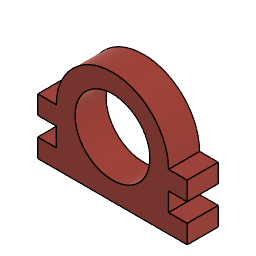
BarrelJackMount_v1 (Autodesk Fusion 360 design; units mm, degrees)
Autodesk Fusion 360 part; units mm, degrees
sketch "Sketch1" plane through (0, 0, 0) normal (0, 1, 0) x (1, 0, 0)
  line L0 (9, 1.5) -> (-9, 1.5) construction
  line L1 (-9, 1.5) -> (-9, -1.5) construction
  line L2 (9, -1.5) -> (9, 1.5) construction
  line L3 (9, 1.5) -> (-9, -1.5) construction
  line L4 (-9, 1.5) -> (9, -1.5) construction
  circle A0 centre (0, -4.5) radius 6
  circle A1 centre (0, -4.5) radius 9
  line L5 (0, 1.5) -> (0, 4.5) construction
  line L6 (0, 0) -> (0, -4.5) construction
  line L7 (-9, 1.5) -> (-9, -1.5)
  line L8 (-9, 1.5) -> (-6.7082, 1.5)
  line L9 (-9, -1.5) -> (-9, -4.5)
  line L10 (6.7082, 1.5) -> (9, 1.5)
  line L11 (9, 1.5) -> (9, -4.5)
  line L12 (-9, -1.5) -> (-12, -1.5)
  line L13 (-12, -1.5) -> (-12, -4.5)
  line L14 (-12, -4.5) -> (-9, -4.5)
  line L15 (-9, 1.5) -> (-12, 1.5)
  line L16 (-12, 1.5) -> (-12, 4.5)
  line L17 (9, 1.5) -> (12, 1.5)
  line L18 (12, 1.5) -> (12, 4.5)
  line L19 (12, 4.5) -> (-12, 4.5)
  line L20 (9, -4.5) -> (12, -4.5)
  line L21 (12, -4.5) -> (12, -1.5)
  line L22 (12, -1.5) -> (9, -1.5)
  dimension "d1" = 18
  dimension "d2" = 3
  dimension "d3" = 12
  dimension "d4" = 18
  dimension "d5" = 3
  dimension "d6" = 3
  dimension "d7" = 3
  dimension "d8" = 3
  dimension "d9" = 3
  dimension "d10" = 3
  dimension "d11" = 3
  dimension "d12" = 3
  dimension "d13" = 3
  constraint horizontal L0
  constraint perpendicular L0 L1
  constraint parallel L1 L2
  constraint coincident L3 L6.start
  constraint coincident L4 L6.start
  constraint coincident L6.start origin
  constraint concentric A0 A1
  constraint midpoint L0 L5.start
  constraint perpendicular L0 L5
  constraint coincident A1 L5.end
  constraint coincident A0.centre A1.centre
  constraint vertical L6
  constraint coincident A1 L8.end
  constraint coincident L0 L8.end
  constraint coincident A1 L9.end
  constraint tangent A1 L9
  constraint coincident A1 L10.start
  constraint coincident L0 L10.start
  constraint coincident A1 L11.end
  constraint tangent A1 L11
  constraint perpendicular L9 L12
  constraint perpendicular L12 L13
  constraint perpendicular L9 L14
  constraint perpendicular L1 L15
  constraint perpendicular L15 L16
  constraint perpendicular L2 L17
  constraint perpendicular L17 L18
  constraint perpendicular L11 L20
  constraint perpendicular L20 L21
  measures "d1" distance of L1.end L2.start
  measures "d2" distance of L0.end L1.end
  measures "d3" diameter of A0
  measures "d4" diameter of A1
  measures "d5" distance of L5.start L5.end
  measures "d6" distance of L1.end L12.end
  measures "d7" distance of L12.end L13.end
  measures "d8" distance of L0.end L15.end
  measures "d9" distance of L15.end L16.end
  measures "d10" distance of L0.start L17.end
  measures "d11" distance of L17.end L18.end
  measures "d12" distance of L11.end L20.end
  measures "d13" distance of L20.end L21.end
extrude "Extrude1" add sketch "Sketch1" along normal blind 5
